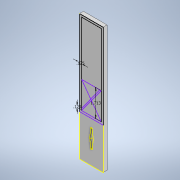
# Autodesk Inventor part: First Leg
Saved by Autodesk Inventor 2020 (Build 240168000, 168)
## iProperties
Created: 2020-03-02
Part Number: First Leg
Material: Generic
Document SubType Name: Modeling
Designer: othscs164
Density: 1 g/cm^3
Appearance: Default
Author: othscs164
Autodesk Inventor part; units mm, degrees
ref_plane "YZ Plane" through (0, 0, 0) normal (1, 0, 0) x (0, 1, 0)
ref_plane "XZ Plane" through (0, 0, 0) normal (0, 1, 0) x (-1, 0, 0)
ref_plane "XY Plane" through (0, 0, 0) normal (0, 0, 1) x (1, 0, 0)
sketch "Sketch1" plane through (0, 0, 0) normal (0, 0, 1) x (1, 0, 0)
  line L0 (0, 0) -> (38.1, 0)
  line L1 (38.1, 0) -> (38.1, 203.2)
  line L2 (38.1, 203.2) -> (0, 203.2)
  line L3 (0, 203.2) -> (0, 0)
  dimension "d0" = 38.1
  dimension "d1" = 203.2
  constraints: 8 end point, 2 parallel, 1 horizontal, 1 perpendicular
  measures "d0" distance of L2.end L1.end
  measures "d1" distance of L1.end L0.end
extrude "Extrusion1" add sketch "Sketch1" along normal blind 6.35
sketch "Sketch2" plane through (0, 0, 6.35) normal (0, 0, 1) x (1, 0, 0)
  line L0 (21.925, 35.9667) -> (21.0447, 23.9538)
  line L1 (17.0553, 23.9538) -> (16.175, 35.9667)
  line L2 (21.925, 40.2333) -> (21.0447, 52.2462)
  line L3 (17.0553, 52.2462) -> (16.175, 40.2333)
  arc A0 (21.925, 35.9667) -> (21.925, 40.2333) centre (19.05, 38.1) ccw
  arc A1 (16.175, 40.2333) -> (16.175, 35.9667) centre (19.05, 38.1) ccw
  arc A2 (17.0553, 23.9538) -> (21.0447, 23.9538) centre (19.05, 24.1) ccw
  arc A3 (21.0447, 52.2462) -> (17.0553, 52.2462) centre (19.05, 52.1) ccw
  line L4 (0, 0) -> (38.1, 0) projected
  line L5 (38.1, 0) -> (38.1, 38.1)
  line L6 (38.1, 0) -> (38.1, 203.2) projected
  line L7 (38.1, 0) -> (76.2, 0) construction
  line L8 (38.1, 38.1) -> (19.05, 38.1)
  line L9 (20.546, 52.2096) -> (21.4374, 40.046)
  arc A4 (21.4374, 36.154) -> (21.4374, 40.046) centre (19.05, 38.1) ccw
  line L10 (21.4374, 36.154) -> (20.546, 23.9904)
  arc A5 (17.554, 23.9904) -> (20.546, 23.9904) centre (19.05, 24.1) ccw
  line L11 (17.554, 23.9904) -> (16.6626, 36.154)
  arc A6 (16.6626, 40.046) -> (16.6626, 36.154) centre (19.05, 38.1) ccw
  line L12 (16.6626, 40.046) -> (17.554, 52.2096)
  arc A7 (20.546, 52.2096) -> (17.554, 52.2096) centre (19.05, 52.1) ccw
  dimension "d4" = 38.1
  dimension "d5" = 90
  dimension "d6" = 19.05
  dimension "d7" = 270
  dimension "d8" = 0.5
  constraints: 22 end point, 16 point on circle, 8 centre point, 2 parallel, 2 perpendicular, 1 collinear, 1 horizontal, 7 other
  measures "d4" distance of L4.end L5.end
  measures "d5" angle of L7 L5
  measures "d6" distance of L5.end L8.end
  measures "d8" distance between parallel lines of L2 L9
extrude "Extrusion2" cut sketch "Sketch2" against normal blind 1.651 contours L9 A4 L10 A5 L11 A6 L12 A7
sketch "Sketch3" plane through (0, 0, 6.35) normal (0, 0, 1) x (1, 0, 0)
  line L0 (21.4374, 36.154) -> (20.546, 23.9904) projected
  arc A0 (17.554, 23.9904) -> (20.546, 23.9904) centre (19.05, 24.1) ccw projected
  line L1 (17.554, 23.9904) -> (16.6626, 36.154) projected
  arc A1 (16.6626, 40.046) -> (16.6626, 36.154) centre (19.05, 38.1) ccw projected
  line L2 (16.6626, 40.046) -> (17.554, 52.2096) projected
  arc A2 (20.546, 52.2096) -> (17.554, 52.2096) centre (19.05, 52.1) ccw projected
  line L3 (20.546, 52.2096) -> (21.4374, 40.046) projected
  arc A3 (21.4374, 36.154) -> (21.4374, 40.046) centre (19.05, 38.1) ccw projected
  line L4 (0, 0) -> (38.1, 0) projected
  line L5 (38.1, 0) -> (38.1, 203.2) projected
  line L6 (38.1, 203.2) -> (0, 203.2) projected
  line L7 (0, 203.2) -> (0, 0) projected
  line L8 (0, 203.2) -> (0, 0) projected
  line L9 (0, 66.3224) -> (38.1, 66.3224)
  line L10 (38.1, 0) -> (38.1, 203.2) projected
  line L11 (0, 66.3224) -> (0, 203.2)
  line L12 (38.1, 203.2) -> (0, 203.2) projected
  line L13 (0, 203.2) -> (38.1, 203.2)
  line L14 (38.1, 203.2) -> (38.1, 66.3224)
  line L15 (3.175, 200.025) -> (3.175, 69.4974)
  line L16 (3.175, 69.4974) -> (34.925, 69.4974)
  line L17 (34.925, 69.4974) -> (34.925, 200.025)
  line L18 (34.925, 200.025) -> (3.175, 200.025)
  line L19 (34.925, 69.4974) -> (34.925, 113.0076)
  line L20 (34.925, 113.0076) -> (3.175, 113.0076)
  line L21 (34.925, 69.4974) -> (3.175, 113.0076)
  line L22 (34.925, 113.0076) -> (3.175, 69.4974)
  line L23 (3.175, 69.4974) -> (19.05, 91.2525)
  line L24 (3.175, 113.0076) -> (19.05, 91.2525)
  line L25 (3.175, 69.4974) -> (3.175, 113.0076)
  line L26 (3.175, 113.0076) -> (34.925, 113.0076)
  line L27 (19.05, 91.2525) -> (34.925, 113.0076)
  line L28 (34.925, 69.4974) -> (19.05, 91.2525)
  line L29 (34.925, 69.4974) -> (34.925, 113.0076)
  line L30 (34.925, 69.4974) -> (3.175, 69.4974)
  line L31 (3.175, 69.4974) -> (3.175, 113.0076)
  line L32 (3.175, 113.0076) -> (34.925, 113.0076)
  line L33 (3.175, 69.4974) -> (3.175, 72.6724)
  line L34 (3.175, 72.6724) -> (32.6082, 113.0076)
  dimension "d12" = 3.175
  dimension "d13" = 43.5102
  dimension "d14" = 3.175
  constraints: 48 end point, 10 perpendicular, 6 point on line, 4 collinear, 1 midpoint, 3 other
  measures "d12" distance between parallel lines of L11 L15
  measures "d13" distance of L16.end L19.end
  measures "d14" distance of L15.end L33.end
body "Solid1"
